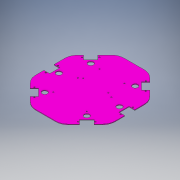
# Autodesk Inventor part: Base
Saved by Autodesk Inventor 2019.1 (Build 231200000, 200)
## iProperties
Created: 2018-10-30
Part Number: Base
Material: Generic
Document SubType Name: Modeling
Designer: kfortuna
Density: 1 g/cm^3
Appearance: Default
Author: kfortuna
Autodesk Inventor part; units mm, degrees
ref_plane "YZ Plane" through (0, 0, 0) normal (1, 0, 0) x (0, 1, 0)
ref_plane "XZ Plane" through (0, 0, 0) normal (0, 1, 0) x (-1, 0, 0)
ref_plane "XY Plane" through (0, 0, 0) normal (0, 0, 1) x (1, 0, 0)
sketch "Sketch1" plane through (0, 0, 0) normal (0, 1, 0) x (-1, 0, 0)
  line L0 (248.9211, 774.0716) -> (204.4366, 774.0716)
  line L1 (204.4366, 574.0727) -> (249.4778, 574.0727)
  line L2 (316.3476, 688.3671) -> (303.3476, 688.3671)
  line L3 (303.3476, 688.3671) -> (303.3476, 665.3671)
  line L4 (303.3476, 665.3671) -> (316.3476, 665.3671)
  line L5 (137.0102, 685.5727) -> (150.0102, 685.5727)
  line L6 (150.0102, 685.5727) -> (150.0102, 662.5836)
  line L7 (150.0102, 662.5836) -> (137.0102, 662.5836)
  line L8 (316.3476, 641.3894) -> (316.3476, 665.3671)
  line L9 (316.3476, 688.3671) -> (316.3476, 706.6452)
  line L10 (137.0102, 706.6452) -> (137.0102, 685.5727)
  line L11 (137.0102, 662.5836) -> (137.0102, 641.4992)
  line L12 (280.7152, 754.704) -> (271.5228, 745.5116)
  line L13 (271.5228, 745.5116) -> (287.7863, 729.2481)
  line L14 (287.7863, 729.2481) -> (296.9787, 738.4405)
  line L15 (158.3637, 607.7192) -> (167.5561, 616.9116)
  line L16 (167.5561, 616.9116) -> (183.8196, 600.6481)
  line L17 (183.8196, 600.6481) -> (174.6272, 591.4557)
  line L18 (145.7969, 620.2859) -> (158.3637, 607.7192)
  line L19 (174.6272, 591.4557) -> (183.2234, 582.8595)
  line L20 (307.5608, 727.8584) -> (296.9787, 738.4405)
  line L21 (280.7152, 754.704) -> (270.1344, 765.2849)
  line L22 (171.0855, 753.147) -> (180.2779, 743.9546)
  line L23 (180.2779, 743.9546) -> (164.0144, 727.6911)
  line L24 (164.0144, 727.6911) -> (154.822, 736.8835)
  line L25 (301.4465, 613.9871) -> (292.1989, 623.1239)
  line L26 (292.1989, 623.1239) -> (276.0337, 606.7628)
  line L27 (276.0337, 606.7628) -> (285.2813, 597.626)
  line L28 (270.8184, 582.9877) -> (285.2813, 597.626)
  line L29 (301.4465, 613.9871) -> (307.6882, 620.3044)
  line L30 (183.2234, 765.2849) -> (171.0855, 753.147)
  line L31 (154.822, 736.8835) -> (145.7969, 727.8584)
  arc A0 (261.9333, 773.4859) -> (260.5191, 774.0716) centre (260.5191, 772.0716) ccw
  arc A1 (270.1344, 765.2849) -> (248.9211, 774.0716) centre (248.9211, 744.0716) ccw
  arc A2 (204.4366, 774.0716) -> (183.2234, 765.2849) centre (204.4366, 744.0716) ccw
  arc A3 (145.7969, 727.8584) -> (137.0102, 706.6452) centre (167.0102, 706.6452) ccw
  arc A4 (137.0102, 641.4992) -> (145.7969, 620.2859) centre (167.0102, 641.4992) ccw
  arc A5 (183.2234, 582.8595) -> (204.4366, 574.0727) centre (204.4366, 604.0727) ccw
  arc A6 (249.4778, 574.0727) -> (270.8184, 582.9877) centre (249.4778, 604.0727) ccw
  arc A7 (307.6882, 620.3044) -> (316.3476, 641.3894) centre (286.3476, 641.3894) ccw
  arc A8 (316.3476, 706.6452) -> (307.5608, 727.8584) centre (286.3476, 706.6452) ccw
  circle A9 centre (279.0199, 600.5369) radius 1.5
  circle A10 centre (309.8476, 663.0421) radius 1.5
  circle A11 centre (309.8476, 690.6921) radius 1.5
  circle A12 centre (294.03, 732.1968) radius 1.5
  circle A13 centre (274.4715, 751.7554) radius 1.5
  circle A14 centre (157.7707, 730.6398) radius 1.5
  circle A15 centre (143.5102, 687.9027) radius 1.5
  circle A16 centre (143.5102, 660.2536) radius 1.5
  circle A17 centre (161.3124, 613.9629) radius 1.5
  circle A18 centre (177.3292, 750.1983) radius 1.5
  circle A19 centre (180.5174, 594.0508) radius 1.5
  circle A20 centre (298.4603, 620.213) radius 1.5
  circle A21 centre (263.158, 720.311) radius 1.25
  circle A22 centre (187.658, 720.311) radius 1.25
  circle A23 centre (263.158, 664.811) radius 1.25
  circle A24 centre (187.658, 664.811) radius 1.25
  line L32 (263.158, 720.311) -> (187.658, 720.311)
  line L33 (263.158, 664.811) -> (187.658, 664.811)
  line L34 (263.158, 720.311) -> (263.158, 664.811)
  line L35 (187.658, 720.311) -> (187.658, 664.811)
  circle A25 centre (256.4035, 659.5938) radius 1.25
  circle A26 centre (199.9035, 659.5938) radius 1.25
  circle A27 centre (256.4035, 623.0938) radius 1.25
  circle A28 centre (199.9035, 623.0938) radius 1.25
  line L36 (256.4035, 659.5938) -> (199.9035, 659.5938)
  line L37 (256.4035, 659.5938) -> (256.4035, 623.0938)
  line L38 (256.4035, 623.0938) -> (199.9035, 623.0938)
  line L39 (199.9035, 623.0938) -> (199.9035, 659.5938)
  circle A29 centre (179.2172, 728.7518) radius 6
  circle A30 centre (160.0102, 674.0836) radius 6
  circle A31 centre (182.7589, 615.8509) radius 6
  circle A32 centre (277.0028, 621.9717) radius 6
  circle A33 centre (294.03, 676.8671) radius 6
  circle A34 centre (272.5835, 730.3088) radius 6
  point P0 (0, 0)
  point P1 (316.3476, 774.0716)
  point P2 (137.0102, 574.0727)
  point P3 (137.0102, 774.0716)
  point P4 (317.0102, 574.0727)
  point P5 (262.0102, 574.0727)
  point P6 (316.3476, 629.0688)
  point P7 (316.3476, 719.0716)
  point P8 (261.3476, 774.0716)
  point P9 (192.0102, 774.0716)
  point P10 (137.0102, 719.0716)
  point P11 (137.0102, 629.0727)
  point P12 (192.0102, 574.0727)
  dimension "d0" = 200
  dimension "d1" = 180
  dimension "d2" = 55
  dimension "d3" = 55
  dimension "d4" = 55
  dimension "d5" = 55
  dimension "d6" = 55
  dimension "d7" = 55
  dimension "d8" = 55
  dimension "d9" = 55
  dimension "d10" = 13
  dimension "d11" = 23
  dimension "d13" = 13
  dimension "d14" = 13
  dimension "d15" = 23
  dimension "d18" = 77.7818
  dimension "d21" = 13
  dimension "d24" = 23
  dimension "d26" = 23
  dimension "d30" = 23
  dimension "d32" = 2
  dimension "d33" = 30
  dimension "d36" = 3
  dimension "d38" = 3
  dimension "d39" = 3
  dimension "d40" = 3
  dimension "d41" = 3
  dimension "d43" = 3
  dimension "d44" = 3
  dimension "d45" = 3
  dimension "d46" = 3
  dimension "d49" = 6.5
  dimension "d50" = 2.325
  dimension "d53" = 2.325
  dimension "d54" = 6.5
  dimension "d55" = 2.33
  dimension "d56" = 6.5
  dimension "d57" = 2.33
  dimension "d58" = 6.5
  dimension "d60" = 3
  dimension "d61" = 6.5
  dimension "d62" = 2.33
  dimension "d63" = 2.33
  dimension "d64" = 6.5
  dimension "d65" = 6.5
  dimension "d66" = 2.33
  dimension "d67" = 6.5
  dimension "d68" = 2.33
  dimension "d69" = 2.33
  dimension "d70" = 6.5
  dimension "d71" = 13
  dimension "d72" = 6
  dimension "d73" = 2.33
  dimension "d74" = 3
  dimension "d75" = 13
  dimension "d78" = 2.33
  dimension "d79" = 6.5
  dimension "d80" = 3
  dimension "d81" = 6.5
  dimension "d82" = 2.33
  dimension "d85" = 9.2476
  dimension "d86" = 13
  dimension "d87" = 13
  dimension "d88" = 13
  constraints: 80 end point, 35 centre point, 24 perpendicular, 22 point on line, 18 point on circle, 18 tangent, 16 parallel, 7 equal radius, 3 horizontal, 1 vertical
  measures "d0" distance of point (317.01, 574.073) point (316.348, 774.072)
  measures "d1" distance of point (137.01, 574.073) point (317.01, 574.073)
  measures "d2" distance of point (262.01, 574.073) point (317.01, 574.073)
  measures "d3" distance of point (316.348, 629.069) point (317.01, 574.073)
  measures "d4" distance of point (316.348, 719.072) point (316.348, 774.072)
  measures "d5" distance of point (261.348, 774.072) point (316.348, 774.072)
  measures "d6" distance of point (192.01, 774.072) point (137.01, 774.072)
  measures "d7" distance of point (137.01, 719.072) point (137.01, 774.072)
  measures "d8" distance of point (137.01, 629.073) point (137.01, 574.073)
  measures "d9" distance of point (192.01, 574.073) point (137.01, 574.073)
  measures "d10" distance of L2.start L2.end
  measures "d11" distance of L2.end L3.end
  measures "d13" distance of L5.start L5.end
  measures "d14" distance of L12.start L12.end
  measures "d15" distance of L12.end L13.end
  measures "d18" distance of point (316.348, 719.072) point (261.348, 774.072)
  measures "d21" distance of L15.start L15.end
  measures "d24" distance between parallel lines of L17 L15
  measures "d26" distance between parallel lines of L24 L22
  measures "d30" distance between parallel lines of L25 L27
  measures "d32" radius of A0
  measures "d33" radius of A1
  measures "d36" diameter of A9
  measures "d38" diameter of A10
  measures "d39" diameter of A11
  measures "d40" diameter of A12
  measures "d41" diameter of A13
  measures "d43" diameter of A14
  measures "d44" diameter of A15
  measures "d45" diameter of A16
  measures "d46" diameter of A17
  measures "d49" distance from line of L8 A10.centre
  measures "d50" distance from line of A10.centre L4
  measures "d53" distance from line of L2 A11.centre
  measures "d54" distance from line of L9 A11.centre
  measures "d55" distance from line of L14 A12.centre
  measures "d56" distance from line of L20 A12.centre
  measures "d57" distance from line of L12 A13.centre
  measures "d58" distance from line of L21 A13.centre
  measures "d60" diameter of A18
  measures "d61" distance from line of L30 A18.centre
  measures "d62" distance from line of L22 A18.centre
  measures "d63" distance from line of L24 A14.centre
  measures "d64" distance from line of L31 A14.centre
  measures "d65" distance from line of L10 A15.centre
  measures "d66" distance from line of L5 A15.centre
  measures "d67" distance from line of L11 A16.centre
  measures "d68" distance from line of L7 A16.centre
  measures "d69" distance from line of L15 A17.centre
  measures "d70" distance from line of L18 A17.centre
  measures "d71" distance between parallel lines of L19 L16
  measures "d72" distance from line of L19 A19.centre
  measures "d73" distance from line of L17 A19.centre
  measures "d74" diameter of A19
  measures "d75" distance of L25.start L25.end
  measures "d78" distance from line of A20.centre L25
  measures "d79" distance from line of L29 A20.centre
  measures "d80" diameter of A20
  measures "d81" distance from line of L28 A9.centre
  measures "d82" distance from line of L27 A9.centre
  measures "d85" horizontal distance of L26.end L27.end
  measures "d86" distance of L6.end L7.end
  measures "d87" distance between parallel lines of L30 L23
  measures "d88" distance between parallel lines of L13 L21
extrude "Extrusion1" add sketch "Sketch1" along normal blind 1.524 contours A1 L21 L12 L13 L14 L20 A8 L9 L2 L3 L4 L8 A7 L29 L25 L26 L27 L28 A6 L1 A5 L19 L17 L16 L15 L18 A4 L11 L7 L6 L5 L10 A3 L31 L24 L23 L22 L30 A2 L0 | A9 | A10 | A11 | A12 | A13 | A14 | A15 | A16 | A17 | A18 | A19 | A20 | A21 L34 L32 | L32 L34 A21 | A21 L34 A23 L33 A24 L35 A22 L32 | L32 L35 A22 | A22 L35 L32 | L34 L33 A23 | A23 L33 L34 | L35 L33 A24 | A24 L33 L35 | A25 L37 L36 | L36 L37 A25 | A25 L37 A27 L38 A28 L39 A26 L36 | L36 L39 A26 | A26 L39 L36 | L37 L38 A27 | A27 L38 L37 | L39 L38 A28 | A28 L38 L39 | A29 | A30 | A31 | A32 | A33 | A34
extrude "Extrusion2" cut sketch "Sketch1" along normal blind 200 contours A9 | A10 | A11 | A12 | A13 | A14 | A15 | A16 | A17 | A18 | A19 | A20
extrude "Extrusion3" cut sketch "Sketch1" along normal blind 200 contours A29 | A30 | A31 | A32 | A33 | A34
extrude "Extrusion5" cut sketch "Sketch1" along normal blind 200 contours A21 L34 L32 | L32 L34 A21 | L32 L35 A22 | A22 L35 L32 | L34 L33 A23 | A23 L33 L34 | L35 L33 A24 | A24 L33 L35 | A25 L37 L36 | L36 L37 A25 | L36 L39 A26 | A26 L39 L36 | L37 L38 A27 | A27 L38 L37 | L39 L38 A28 | A28 L38 L39
equation "\"d3\" = d2"
equation "\"d5\" = d4"
equation "\"d6\" = d4"
equation "\"d7\" = d6"
equation "\"d8\" = d4"
equation "\"d9\" = d8"
body "Solid1"
